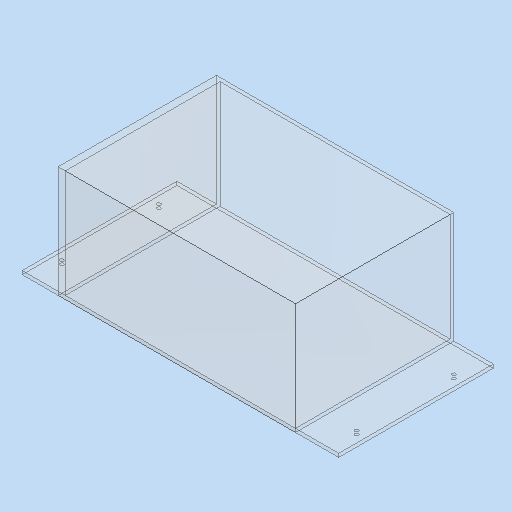
# Autodesk Inventor part: Proteção de acrilico
Saved by Autodesk Inventor 2026.2 (Build 302298010, 298A)
## iProperties
Created: 2026-05-23
Part Number: Proteção de acrilico
Material: Generic
Document SubType Name: Modeling
Designer: Rubens
Density: 1 g/cm^3
Appearance: Polycarbonate - Clear
Author: Rubens
Autodesk Inventor part; units mm, degrees
ref_plane "YZ Plane" through (0, 0, 0) normal (1, 0, 0) x (0, 1, 0)
ref_plane "XZ Plane" through (0, 0, 0) normal (0, 1, 0) x (-1, 0, 0)
ref_plane "XY Plane" through (0, 0, 0) normal (0, 0, 1) x (1, 0, 0)
sketch "Sketch1" plane through (0, 0, 0) normal (0, 0, 1) x (1, 0, 0)
  line L0 (0, 0) -> (440, 0)
  line L1 (220, 0) -> (380, 0)
  line L2 (220, 0) -> (60, 0)
  line L3 (60, 2.9881) -> (60, 155)
  line L4 (60, 155) -> (380, 155)
  line L5 (380, 155) -> (380, 0)
  line L6 (60, -5) -> (220, -5)
  line L7 (220, -5) -> (385, -5)
  line L8 (385, -5) -> (385, 160)
  line L9 (385, 160) -> (55, 160)
  line L10 (55, 160) -> (55, 2.9881)
  line L11 (0, 0) -> (0, 5)
  line L12 (0, 5) -> (440, 5)
  line L13 (440, 5) -> (440, 0)
  point P0 (385, 5)
  point P1 (55, 5)
  point P2 (380, 5)
  point P3 (60, 5)
  dimension "d0" = 440
  dimension "d1" = 160
  dimension "d2" = 160
  dimension "d4" = 5
  dimension "d5" = 5
  dimension "d16" = 150
  constraints: 28 end point, 3 perpendicular, 2 horizontal, 2 point on line, 2 vertical, 1 midpoint, 1 parallel, 4 other
  measures "d0" distance of L0.start L0.end
  measures "d1" distance of L1.start L1.end
  measures "d2" distance of L1.start L2.end
  measures "d4" distance between parallel lines of L4 L9
  measures "d5" distance of L0.start L11.end
  measures "d16" distance between parallel lines of L12 L4
extrude "Extrusion1" add sketch "Sketch1" against normal blind 215 contours L11 L12 L5 L0 | L10 L9 L8 L12 L5 L4 L3 | L5 L12 L8 L0 | L8 L12 L13 L0
sketch "Sketch2" plane through (0, 5, 0) normal (0, 1, 0) x (1, 0, 0)
  line L0 (0, 0) -> (0, 215) projected
  line L1 (0, 215) -> (15, 215)
  line L2 (440, 215) -> (0, 215) projected
  line L3 (15, 215) -> (15, -133.1496)
  line L4 (440, 215) -> (425, 215)
  line L5 (425, 215) -> (425, -133.1496)
  circle A0 centre (15, 175) radius 2.5
  circle A1 centre (15, 40) radius 2.5
  line L6 (55, 0) -> (0, 0) projected
  line L7 (220, 215) -> (220, -93.5309)
  circle A2 centre (425, 175) radius 2.5
  circle A3 centre (425, 40) radius 2.5
  dimension "d8" = 15
  dimension "d9" = 15
  dimension "d10" = 5
  dimension "d11" = 5
  dimension "d12" = 40
  dimension "d13" = 40
  constraints: 10 end point, 4 centre point, 4 point on line, 2 perpendicular, 2 symmetric about line, 1 midpoint, 1 vertical, 2 other
  measures "d8" distance of L0.end L1.end
  measures "d9" distance of L2.start L4.end
  measures "d10" diameter of A0
  measures "d11" diameter of A1
  measures "d12" distance from line of L2 A0.centre
  measures "d13" distance from line of L6 A1.centre
extrude "Extrusion2" cut sketch "Sketch2" against normal blind 215 contours A3 L5 | L5 A3 | A2 L5 | L5 A2 | A1 L3 | L3 A1 | A0 L3 | L3 A0
sketch "Sketch3" plane through (0, 0, 0) normal (0, 0, 1) x (1, 0, 0)
  line L0 (0, 5) -> (55, 5) projected
  line L1 (55, 160) -> (385, 160) projected
  line L2 (55, 5) -> (385, 5)
  line L3 (385, 5) -> (385, 160)
  line L4 (385, 160) -> (55, 160)
  line L5 (55, 160) -> (55, 5)
  point P0 (0, 0)
  constraints: 8 end point, 2 parallel, 1 horizontal, 1 perpendicular
extrude "Extrusion3" add sketch "Sketch3" along normal blind 5
body "Solid1"
